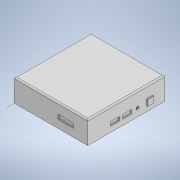
# Autodesk Inventor part: NUC_model
Saved by Autodesk Inventor 2020 (Build 240168000, 168)
## iProperties
Created: 2019-07-08
Part Number: NUC_model
Material: Generic
Document SubType Name: Modeling
Designer: Senior Design
Density: 1 g/cm^3
Appearance: Default
Author: Senior Design
Autodesk Inventor part; units mm, degrees
ref_plane "YZ Plane" through (0, 0, 0) normal (1, 0, 0) x (0, 1, 0)
ref_plane "XZ Plane" through (0, 0, 0) normal (0, 1, 0) x (-1, 0, 0)
ref_plane "XY Plane" through (0, 0, 0) normal (0, 0, 1) x (1, 0, 0)
sketch "Sketch1" plane through (0, 0, 0) normal (0, 1, 0) x (-1, 0, 0)
  line L0 (55.925, 58.5) -> (-55.925, 58.5)
  line L1 (-55.925, 58.5) -> (-55.925, -58.5)
  line L2 (-55.925, -58.5) -> (55.925, -58.5)
  line L3 (55.925, -58.5) -> (55.925, 58.5)
  line L4 (55.925, 58.5) -> (-55.925, -58.5) construction
  line L5 (-55.925, 58.5) -> (55.925, -58.5) construction
  point P0 (0, 0)
  dimension "d0" = 111.85
  dimension "d1" = 117
  constraints: 12 end point, 2 midpoint, 2 parallel, 1 horizontal, 1 perpendicular
  measures "d0" distance of L0.start L0.end
  measures "d1" distance of L0.end L1.end
extrude "Extrusion1" add sketch "Sketch1" along normal blind 34.19
fillet "Fillet1" radius 2 4 edges at (0, 34.19, 58.5) (55.925, 34.19, 0) (0, 34.19, -58.5) (-55.925, 34.19, 0)
sketch "Sketch2" plane through (0, 0, 0) normal (0, -1, 0) x (1, 0, 0)
  circle A0 centre (45.425, 48) radius 5.375
  line L0 (55.925, 58.5) -> (55.925, -58.5) projected
  line L1 (-55.925, 58.5) -> (55.925, 58.5) projected
  circle A1 centre (-45.575, 48) radius 5.375
  circle A2 centre (45.425, -47) radius 5.375
  circle A3 centre (-45.575, -47) radius 5.375
  point P0 (0, 0)
  dimension "d5" = 10.75
  dimension "d6" = 10.5
  dimension "d7" = 10.5
  dimension "d10" = 91
  dimension "d13" = 95
  constraints: 4 centre point, 1 horizontal, 1 vertical, 6 other
  measures "d5" diameter of A0
  measures "d6" distance from line of L0 A0.centre
  measures "d7" distance from line of L1 A0.centre
  measures "d10" distance of A0.centre A1.centre
  measures "d13" distance of A0.centre A2.centre
extrude "Extrusion2" add sketch "Sketch2" along normal blind 1.5
sketch "Sketch4" plane through (0, 0, 0) normal (0, -1, 0) x (1, 0, 0)
  line L0 (-55.925, -58.5) -> (-55.925, 58.5) projected
  line L1 (-55.925, 58.5) -> (55.925, 58.5) projected
  point P0 (0, 0)
  point P1 (-42.625, 0)
  dimension "d32" = 13.3
  dimension "d33" = 58.5
  measures "d32" distance from line of L0 point (-42.625, 0)
  measures "d33" distance from line of L1 point (-42.625, 0)
hole "Hole2" at (-42.625, 0, 0) direction (0, 1, 0) diameter 3 depth 1 tip angle 118
pattern_linear "Rectangular Pattern1" count 2 spacing 84.5 along (1, 0, 0) of "Hole2"
sketch "Sketch5" plane through (55.925, 0, 58.5) normal (1, 0, 0) x (0, 0, -1)
  line L0 (34.3, 14.5) -> (47.9, 14.5)
  line L1 (47.9, 14.5) -> (47.9, 8.6)
  line L2 (47.9, 8.6) -> (34.3, 8.6)
  line L3 (34.3, 8.6) -> (34.3, 14.5)
  line L4 (34.3, 14.5) -> (47.9, 8.6) construction
  line L5 (47.9, 14.5) -> (34.3, 8.6) construction
  line L6 (52.76, 14.5) -> (66.36, 14.5)
  line L7 (66.36, 14.5) -> (66.36, 8.6)
  line L8 (66.36, 8.6) -> (52.76, 8.6)
  line L9 (52.76, 8.6) -> (52.76, 14.5)
  line L10 (52.76, 14.5) -> (66.36, 8.6) construction
  line L11 (66.36, 14.5) -> (52.76, 8.6) construction
  line L12 (0, 0) -> (117, 0) projected
  line L13 (0, 0) -> (0, 32.19) projected
  point P0 (58.5, 0)
  point P1 (41.1, 11.55)
  point P2 (59.56, 11.55)
  dimension "d37" = 13.6
  dimension "d38" = 5.9
  dimension "d39" = 13.6
  dimension "d40" = 5.9
  dimension "d41" = 8.6
  dimension "d42" = 34.3
  dimension "d43" = 4.86
  dimension "d44" = 8.6
  constraints: 24 end point, 4 midpoint, 4 parallel, 2 horizontal, 2 perpendicular
  measures "d37" distance of L1.end L2.end
  measures "d38" distance of L0.end L1.end
  measures "d39" distance of L8.start L9.start
  measures "d40" distance of L6.end L8.start
  measures "d41" distance between parallel lines of L12 L2
  measures "d42" distance between parallel lines of L13 L3
  measures "d43" distance between parallel lines of L9 L1
  measures "d44" distance between parallel lines of L8 L12
extrude "Extrusion3" cut sketch "Sketch5" against normal blind 1.5
sketch "Sketch6" plane through (55.925, 0, 58.5) normal (1, 0, 0) x (0, 0, -1)
  line L0 (66.36, 14.5) -> (66.36, 8.6) projected
  line L1 (0, 0) -> (117, 0) projected
  point P0 (58.5, 0)
  point P1 (75.26, 12)
  dimension "d54" = 8.9
  dimension "d55" = 12
  measures "d54" distance from line of L0 point (75.26, 12)
  measures "d55" distance from line of L1 point (75.26, 12)
hole "Hole3" at (55.925, 12, -16.76) direction (-1, 0, 0) diameter 4.24 depth 10.688 tip angle 118
sketch "Sketch7" plane through (-55.925, 0, -58.5) normal (-1, 0, 0) x (0, 0, 1)
  line L0 (0, 0) -> (117, 0) projected
  line L1 (0, 0) -> (0, 32.19) projected
  point P0 (58.5, 0)
  point P1 (20, 9.25)
  dimension "d56" = 9.25
  dimension "d64" = 20
  measures "d56" distance from line of L0 point (20, 9.25)
  measures "d64" distance from line of L1 point (20, 9.25)
hole "Hole4" at (-55.925, 9.25, -38.5) direction (1, 0, 0) diameter 6.88 depth 10.688 tip angle 118
sketch "Sketch8" plane through (-55.925, 0, -58.5) normal (-1, 0, 0) x (0, 0, 1)
  line L0 (33.6837, 13.1926) -> (42.498, 13.1926)
  line L1 (46.62, 11.6426) -> (46.62, 8.31)
  line L2 (46.62, 8.31) -> (30.5, 8.31)
  line L3 (30.5, 8.31) -> (30.5, 11.6426)
  line L4 (30.5, 14.87) -> (46.62, 8.31) construction
  line L5 (46.62, 14.87) -> (30.5, 8.31) construction
  circle A0 centre (20, 9.25) radius 3.44 projected
  line L6 (0, 0) -> (117, 0) projected
  line L7 (30.5, 11.6426) -> (33.6837, 13.1926)
  line L8 (42.498, 13.1926) -> (46.62, 11.6426)
  point P0 (58.5, 0)
  point P1 (38.56, 11.59)
  dimension "d65" = 16.12
  dimension "d66" = 6.56
  dimension "d67" = 10.5
  dimension "d68" = 8.31
  dimension "d69" = 1.55
  dimension "d70" = 1.55
  dimension "d71" = 8.8143
  constraints: 16 end point, 2 midpoint, 2 parallel, 1 horizontal, 1 perpendicular, 1 point on line
  measures "d65" distance of L4.start L5.start
  measures "d66" distance of L5.start L1.end
  measures "d67" distance from line of A0.centre L3
  measures "d68" distance between parallel lines of L6 L2
  measures "d69" vertical distance of L0.start L3.end
  measures "d70" vertical distance of L1.start L0.end
  measures "d71" distance of L0.end L0.start
extrude "Extrusion4" cut sketch "Sketch8" against normal blind 1.5 contours L0 L8 L1 L2 L3 L7
sketch "Sketch10" plane through (-55.925, 0, -58.5) normal (-1, 0, 0) x (0, 0, 1)
  line L0 (51.62, 18.8) -> (67.17, 18.8)
  line L1 (67.17, 18.8) -> (67.17, 7.1)
  line L2 (67.17, 7.1) -> (51.62, 7.1)
  line L3 (51.62, 7.1) -> (51.62, 18.8)
  line L4 (51.62, 18.8) -> (67.17, 7.1) construction
  line L5 (67.17, 18.8) -> (51.62, 7.1) construction
  line L6 (46.62, 11.6426) -> (46.62, 8.31) projected
  line L7 (0, 0) -> (117, 0) projected
  point P0 (58.5, 0)
  point P1 (59.395, 12.95)
  dimension "d81" = 15.55
  dimension "d82" = 11.7
  dimension "d84" = 5
  dimension "d85" = 7.1
  constraints: 12 end point, 2 midpoint, 2 parallel, 1 horizontal, 1 perpendicular
  measures "d81" distance of L1.end L2.end
  measures "d82" distance of L0.end L1.end
  measures "d84" distance between parallel lines of L3 L6
  measures "d85" distance between parallel lines of L7 L2
extrude "Extrusion5" cut sketch "Sketch10" against normal blind 1.5
sketch "Sketch11" plane through (-55.925, 0, -58.5) normal (-1, 0, 0) x (0, 0, 1)
  line L0 (71.57, 20.05) -> (85.87, 20.05)
  line L1 (85.87, 20.05) -> (85.87, 13.45)
  line L2 (85.87, 13.45) -> (71.57, 13.45)
  line L3 (71.57, 13.45) -> (71.57, 20.05)
  line L4 (71.57, 20.05) -> (85.87, 13.45) construction
  line L5 (85.87, 20.05) -> (71.57, 13.45) construction
  line L6 (0, 32.19) -> (117, 32.19) projected
  line L7 (67.17, 18.8) -> (67.17, 7.1) projected
  line L8 (71.57, 11.05) -> (85.87, 11.05)
  line L9 (85.87, 11.05) -> (85.87, 4.45)
  line L10 (85.87, 4.45) -> (71.57, 4.45)
  line L11 (71.57, 4.45) -> (71.57, 11.05)
  point P0 (58.5, 0)
  point P1 (78.72, 16.75)
  point P2 (79.72, 17.75)
  dimension "d88" = 14.3
  dimension "d89" = 6.6
  dimension "d90" = 12.14
  dimension "d91" = 4.4
  dimension "d92" = 14.3
  dimension "d93" = 6.6
  dimension "d94" = 2.4
  dimension "d95" = 4.4
  constraints: 20 end point, 4 parallel, 2 horizontal, 2 midpoint, 2 perpendicular
  measures "d88" distance of L1.end L2.end
  measures "d89" distance of L0.end L1.end
  measures "d90" distance between parallel lines of L6 L0
  measures "d91" distance between parallel lines of L3 L7
  measures "d92" distance of L9.end L11.start
  measures "d93" distance of L8.end L9.end
  measures "d94" distance between parallel lines of L8 L2
  measures "d95" distance between parallel lines of L7 L11
extrude "Extrusion6" cut sketch "Sketch11" against normal blind 1.5
sketch "Sketch12" plane through (-55.925, 0, -58.5) normal (-1, 0, 0) x (0, 0, 1)
  line L0 (93.15, 19.5997) -> (99.7593, 19.5997) construction
  line L1 (93.15, 17.8293) -> (99.7593, 17.8293)
  line L2 (99.7593, 21.37) -> (93.15, 21.37)
  arc A0 (93.15, 21.37) -> (93.15, 17.8293) centre (93.15, 19.5997) ccw
  arc A1 (99.7593, 17.8293) -> (99.7593, 21.37) centre (99.7593, 19.5997) ccw
  line L3 (0, 32.19) -> (117, 32.19) projected
  line L4 (85.87, 20.05) -> (85.87, 13.45) projected
  point P0 (58.5, 0)
  point P1 (96.4547, 19.5997)
  dimension "d98" = 10.15
  dimension "d99" = 10.82
  dimension "d100" = 7.28
  constraints: 8 end point, 4 point on circle, 4 tangent, 2 centre point, 1 horizontal, 1 midpoint, 1 parallel
  measures "d99" distance between parallel lines of L3 L2
  measures "d100" distance from line of L4 L0.start
extrude "Extrusion7" cut sketch "Sketch12" against normal blind 1.5
sketch "Sketch13" plane through (55.925, 0, 58.5) normal (1, 0, 0) x (0, 0, -1)
  line L0 (89.56, 16.8) -> (98.76, 16.8)
  line L1 (98.76, 16.8) -> (98.76, 7.6)
  line L2 (98.76, 7.6) -> (89.56, 7.6)
  line L3 (89.56, 7.6) -> (89.56, 16.8)
  line L4 (89.56, 16.8) -> (98.76, 7.6) construction
  line L5 (98.76, 16.8) -> (89.56, 7.6) construction
  circle A0 centre (75.26, 12) radius 2.12 projected
  line L6 (0, 0) -> (117, 0) projected
  point P0 (58.5, 0)
  point P1 (94.16, 12.2)
  dimension "d103" = 14.3
  dimension "d104" = 7.6
  dimension "d105" = 9.2
  dimension "d106" = 9.2
  constraints: 12 end point, 2 midpoint, 2 parallel, 1 horizontal, 1 perpendicular
  measures "d103" distance from line of L3 A0.centre
  measures "d104" distance between parallel lines of L6 L2
  measures "d105" distance of L0.start L0.end
  measures "d106" distance of L0.end L1.end
extrude "Extrusion8" add sketch "Sketch13" along normal blind 1.5 contours L0 L1 L2 L3
sketch "Sketch14" plane through (-55.925, 0, 58.5) normal (0, 0, 1) x (1, 0, 0)
  line L0 (66.65, 18.82) -> (90.15, 18.82)
  line L1 (90.15, 18.82) -> (90.15, 12.25)
  line L2 (90.15, 12.25) -> (66.65, 12.25)
  line L3 (66.65, 12.25) -> (66.65, 18.82)
  line L4 (66.65, 18.82) -> (90.15, 12.25) construction
  line L5 (90.15, 18.82) -> (66.65, 12.25) construction
  line L6 (0, 0) -> (111.85, 0) projected
  line L7 (111.85, 0) -> (111.85, 32.19) projected
  point P0 (55.925, 0)
  point P1 (78.4, 15.535)
  dimension "d109" = 23.5
  dimension "d110" = 6.57
  dimension "d111" = 12.25
  dimension "d112" = 21.7
  constraints: 12 end point, 2 midpoint, 2 parallel, 1 horizontal, 1 perpendicular
  measures "d109" distance of L1.end L2.end
  measures "d110" distance of L0.end L1.end
  measures "d111" distance between parallel lines of L6 L2
  measures "d112" distance between parallel lines of L7 L1
extrude "Extrusion9" cut sketch "Sketch14" against normal blind 1.5
body "Solid1"
